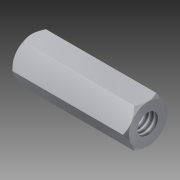
# Autodesk Inventor part: 0.75 inch Standoff
Saved by Autodesk Inventor 2016 SP2 (Build 200236200, 236)
## iProperties
Company: Autodesk Inc.
Category: Structure
Part Number: 0.75 inch Standoff
Document SubType Name: Modeling
Designer: Autodesk Inc.
Material: Steel
Mass: 12.1643 g
Surface Area: 14.4684 cm^2
Volume: 1.54959 cm^3
Density: 7.85 g/cm^3
Created: 2012-04-12
Catalog Web Link: http://www.vexrobotics.com/standoffs-8-32.html
Vendor: VEX
Appearance: Aluminum - Flat
Author: Autodesk Inc.
Autodesk Inventor part; units mm, degrees
ref_plane "YZ Plane" through (0, 0, 0) normal (1, 0, 0) x (0, 1, 0)
sketch "Sketch1" plane through (0, 0, 0) normal (0, 0, 1) x (1, 0, 0)
  line L0 (1.9552, -3.1747) -> (-1.711, -3.1747)
  line L1 (-1.711, -3.1747) -> (-3.5441, 0.0003)
  line L2 (-3.5441, 0.0003) -> (-1.711, 3.1753)
  line L3 (-1.711, 3.1753) -> (1.9552, 3.1753)
  line L4 (1.9552, 3.1753) -> (3.7883, 0.0003)
  line L5 (3.7883, 0.0003) -> (1.9552, -3.1747)
  point P0 (0.1221, 0.0003)
  dimension "d0" = 6.35
  constraints: 12 end point, 1 horizontal, 11 other
  measures "d0" distance between parallel lines of L0 L3
extrude "Extrusion1" add sketch "Sketch1" along normal blind 19.05
ref_plane "Work Plane1" through (-1.711, 0.0003, 0) normal (0, 1, 0) x (1, 0, 0)
sketch "Sketch3" plane through (-1.711, 0.0003, 0) normal (0, 1, 0) x (1, 0, 0)
  line L0 (-1.3251, 0) -> (4.9741, 0)
  line L1 (5.4821, -0.508) -> (5.4821, -18.542)
  line L2 (-1.8331, -18.542) -> (-1.8331, -0.508)
  line L3 (-1.8331, -0.508) -> (-1.3251, 0)
  line L4 (4.9741, 0) -> (5.4821, -0.508)
  line L5 (-1.8331, 0) -> (-1.8331, -19.05) projected
  line L6 (3.6662, 0) -> (5.4993, 0) projected
  line L7 (1.8245, 0) -> (1.8245, -19.05)
  line L8 (0, -19.05) -> (-1.8331, -19.05) projected
  line L9 (5.4993, -19.05) -> (3.6662, -19.05) projected
  line L10 (3.6662, -19.05) -> (0, -19.05) projected
  line L11 (-1.3251, -19.05) -> (-1.8331, -18.542)
  line L12 (4.9741, -19.05) -> (5.4821, -18.542)
  point P0 (-1.8331, 0)
  point P1 (5.4821, 0)
  point P2 (5.4821, -19.05)
  dimension "d5" = 0.508
  dimension "d6" = 0.508
  dimension "d7" = 0.508
  dimension "d8" = 0.508
  dimension "d16" = 0
  dimension "d46" = 0.508
  dimension "d47" = 0.508
  dimension "d48" = 0.508
  dimension "d49" = 0.508
  constraints: 16 end point, 9 point on line, 2 parallel, 2 perpendicular, 1 horizontal, 1 midpoint
  measures "d5" distance of L2.end point (-1.833, 0)
  measures "d6" distance of L0.start point (-1.833, 0)
  measures "d7" distance of L0.end point (5.482, 0)
  measures "d8" distance of L1.start point (5.482, 0)
  measures "d16" distance between parallel lines of L0 L6
  measures "d46" horizontal distance of L11.start L2.start
  measures "d47" horizontal distance of L11.start L2.start
  measures "d48" horizontal distance of L12.start L1.end
  measures "d49" horizontal distance of L12.start L1.end
revolve "Revolution1" cut sketch "Sketch3" angle 360 about axis through (0.1135, 0.0003, 0) along (0, 0, 1) keep common part contours L0 L4 L1 L12 L9 L10 L7
sketch "Sketch6" plane through (0.1135, 0.0003, 0) normal (0, 0, -1) x (-1, 0, 0)
  circle A0 centre (0, 0) radius 3.1496 projected
  constraints: 1 coincident
hole "Hole3" at (0.1135, 0.0003, 0) direction (0, 0, 1) diameter 3.302 depth 6.35 tip angle 118 thread size "8-32 UNC" class "2B" standard "ANSI Unified Screw Threads"
sketch "Sketch7" plane through (0, 0, 19.05) normal (0, 0, 1) x (1, 0, 0)
  point P0 (0, 0)
hole "Hole4" at (0, 0, 19.05) direction (0, 0, -1) diameter 3.302 depth 6.35 tip angle 118 thread size "8-32 UNC" class "2B" standard "ANSI Unified Screw Threads"
ref_plane "Work Plane2" through (0.1135, 0.0003, 9.525) normal (0, 0, -1) x (-1, 0, 0)
equation "\"d6\" = d5"
equation "\"d7\" = d5"
equation "\"d8\" = d7"
body "Solid1"
